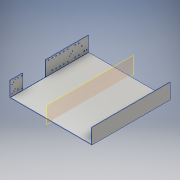
# Autodesk Inventor part: SheetBottomFloorV01saved01
Saved by Autodesk Inventor 2016 SP1 (Build 200210100, 210)
## iProperties
Created: 2016-02-09
Part Number: SheetBottomFloorV01saved01
Material: Aluminum 6061
Document SubType Name: Modeling
Designer: steele
Density: 2.7 g/cm^3
Appearance: Aluminum - Flat
Author: steele
Autodesk Inventor part; units mm, degrees
ref_plane "XZ Plane" through (0, 0, 0) normal (0, 1, 0) x (-1, 0, 0)
ref_plane "XY Plane" through (0, 0, 0) normal (0, 0, 1) x (1, 0, 0)
sketch "Sketch1" plane through (0, 0, 0) normal (0, 0, 1) x (1, 0, 0)
  line L0 (0, 0) -> (-273.05, 0)
  line L1 (-273.05, 0) -> (-273.05, 101.6)
  line L2 (-273.05, 101.6) -> (-269.875, 101.6)
  line L3 (-269.875, 101.6) -> (-269.875, 3.175)
  line L4 (0, 0) -> (0, 3.175) construction
  line L5 (0, 3.175) -> (-269.875, 3.175)
  line L6 (0, 0) -> (273.05, 0)
  line L7 (273.05, 0) -> (273.05, 101.6)
  line L8 (273.05, 101.6) -> (269.875, 101.6)
  line L9 (269.875, 101.6) -> (269.875, 3.175)
  line L10 (0, 3.175) -> (269.875, 3.175)
  dimension "d0" = 101.6
  dimension "d1" = 273.05
  dimension "d2" = 3.175
  dimension "d4" = 3.175
  constraints: 22 end point, 4 symmetric about line, 2 horizontal, 2 perpendicular, 1 parallel, 1 vertical
  measures "d0" distance of L0.end L1.end
  measures "d1" distance of L0.start L0.end
  measures "d2" distance between parallel lines of L1 L3
  measures "d4" distance of L0.start L4.end
extrude "Extrusion1" add sketch "Sketch1" along normal mid plane 520.7
fillet "Fillet1" radius 0.7937 2 edges at (-269.875, 3.175, 0) (269.875, 3.175, 0)
sketch "Sketch5" plane through (-269.875, 101.6, 260.35) normal (1, 0, 0) x (0, 0, -1)
  circle A0 centre (12.7, -30.1625) radius 2.5527 projected
  circle A1 centre (22.225, -20.6375) radius 2.5527 projected
  circle A2 centre (31.75, -11.1125) radius 2.5527 projected
  circle A3 centre (50.8, -11.1125) radius 3.3782 projected
  circle A4 centre (76.2, -11.1125) radius 3.7287 projected
  circle A5 centre (12.7, -84.1375) radius 2.667 projected
  circle A6 centre (22.225, -74.6125) radius 2.667 projected
  circle A7 centre (31.75, -65.0875) radius 2.5527 projected
  circle A8 centre (50.8, -77.7875) radius 3.8163 projected
  circle A9 centre (76.2, -84.1375) radius 3.3782 projected
  circle A10 centre (101.4806, -88.9127) radius 3.3782 projected
  circle A11 centre (212.631, -88.9127) radius 3.3782 projected
  circle A12 centre (228.6, -84.1375) radius 3.7287 projected
  circle A13 centre (279.4, -81.5975) radius 3.8163 projected
  circle A14 centre (228.6, -11.1125) radius 3.3782 projected
  circle A15 centre (254, -11.1125) radius 3.7287 projected
  circle A16 centre (279.4, -11.1125) radius 3.3782 projected
  circle A17 centre (304.8, -11.1125) radius 3.3782 projected
  circle A18 centre (330.2, -11.1125) radius 3.7287 projected
  circle A19 centre (355.6, -11.1125) radius 3.3782 projected
  circle A20 centre (381, -11.1125) radius 3.3782 projected
  circle A21 centre (431.8, -11.1125) radius 3.7287 projected
  circle A22 centre (454.025, -14.2875) radius 3.8163 projected
  circle A23 centre (508, -77.7875) radius 3.8163 projected
  circle A24 centre (457.2, -84.1375) radius 3.3782 projected
  circle A25 centre (431.8, -84.1375) radius 3.7287 projected
  circle A26 centre (475.0995, -39.081) radius 3.3782 projected
  circle A27 centre (412.75, -38.1) radius 2.5527 projected
  circle A28 centre (403.225, -47.625) radius 2.667 projected
  circle A29 centre (393.7, -57.15) radius 2.5527 projected
  circle A30 centre (381, -84.1375) radius 3.3782 projected
  circle A31 centre (355.6, -84.1375) radius 3.3782 projected
  circle A32 centre (330.2, -84.1375) radius 3.7287 projected
  circle A33 centre (304.8, -84.1375) radius 3.3782 projected
  circle A34 centre (492.125, -77.7875) radius 4.826 projected
  circle A35 centre (508, -77.7875) radius 5.2255 projected
  point P0 (260.35, -101.6)
extrude "Extrusion2" cut sketch "Sketch5" against normal through all contours A0 | A1 | A2 | A3 | A4 | A5 | A6 | A7 | A8 | A9 | A10 | A11 | A12 | A13 | A14 | A15 | A16 | A17 | A18 | A19 | A20 | A21 | A22 | A23 | A24 | A25 | A26 | A27 | A28 | A29 | A30 | A31 | A32 | A33 | A34
sketch "Sketch6" plane through (-269.875, 101.6, 260.35) normal (1, 0, 0) x (0, 0, -1)
  line L0 (0, 0) -> (520.7, 0) projected
  line L1 (0, -101.6) -> (520.7, -101.6) projected
  line L2 (82.55, 0) -> (234.95, 0)
  line L3 (234.95, 0) -> (234.95, -101.6)
  line L4 (234.95, -101.6) -> (82.55, -101.6)
  line L5 (82.55, -101.6) -> (82.55, 0)
  line L6 (0, 0) -> (0, -101.6) projected
  point P0 (260.35, -101.6)
  dimension "d18" = 82.55
  dimension "d19" = 234.95
  constraints: 8 end point, 2 parallel, 2 point on line, 1 horizontal, 1 perpendicular
  measures "d18" distance between parallel lines of L6 L5
  measures "d19" distance between parallel lines of L3 L6
extrude "Extrusion3" cut sketch "Sketch6" against normal through all contours L0 L3 L1 L5
body "Solid1"
